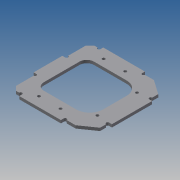
# Autodesk Inventor part: refuerzo interior B
Saved by Autodesk Inventor 2017 (Build 210142000, 142)
## iProperties
Part Number: refuerzo interior B
Material: Genérico
Document SubType Name: Modeling
Designer: Leo
Density: 1 g/cm^3
Appearance: Valor por defecto
Description: Aluminio compuesto routeado CNC
Author: Leo
Autodesk Inventor part; units mm, degrees
ref_plane "YZ Plane" through (0, 0, 0) normal (1, 0, 0) x (0, 1, 0)
ref_plane "XZ Plane" through (0, 0, 0) normal (0, 1, 0) x (-1, 0, 0)
ref_plane "XY Plane" through (0, 0, 0) normal (0, 0, 1) x (1, 0, 0)
sketch "Boceto1" plane through (0, 0, 0) normal (0, 0, 1) x (1, 0, 0)
  line L0 (0, 82.4534) -> (0, -82.4534) construction
  line L1 (-81.8976, 0) -> (81.8976, 0) construction
  line L2 (54.5, 40.5) -> (54.5, 32)
  arc A0 (54.5, 32) -> (54.5, 28) centre (54.5, 30) ccw
  line L3 (54.5, 28) -> (58.5, 28)
  line L4 (58.5, 28) -> (58.5, -28)
  line L5 (58.5, -28) -> (54.5, -28)
  arc A1 (54.5, -28) -> (54.5, -32) centre (54.5, -30) ccw
  line L6 (54.5, -32) -> (54.5, -40.5)
  line L7 (-54.5, 48.5) -> (-54.5, 24)
  arc A2 (-54.5, 20) -> (-54.5, 24) centre (-54.5, 22) ccw
  line L8 (-54.5, 20) -> (-58.5, 20)
  line L9 (-58.5, 20) -> (-58.5, -20)
  line L10 (-58.5, -20) -> (-54.5, -20)
  arc A3 (-54.5, -24) -> (-54.5, -20) centre (-54.5, -22) ccw
  line L11 (-54.5, -24) -> (-54.5, -48.5)
  line L12 (-48.5, 54.5) -> (-44, 54.5)
  line L13 (22, 54.5) -> (34.5, 54.5)
  line L14 (-48.5, -54.5) -> (-44, -54.5)
  line L15 (22, -54.5) -> (34.5, -54.5)
  arc A4 (-44, 54.5) -> (-40, 54.5) centre (-42, 54.5) ccw
  line L16 (-40, 54.5) -> (-40, 58.5)
  line L17 (-40, 58.5) -> (18, 58.5)
  line L18 (18, 58.5) -> (18, 54.5)
  arc A5 (18, 54.5) -> (22, 54.5) centre (20, 54.5) ccw
  arc A6 (-40, -54.5) -> (-44, -54.5) centre (-42, -54.5) ccw
  line L19 (-40, -54.5) -> (-40, -58.5)
  line L20 (-40, -58.5) -> (18, -58.5)
  line L21 (18, -58.5) -> (18, -54.5)
  arc A7 (22, -54.5) -> (18, -54.5) centre (20, -54.5) ccw
  line L22 (-54.5, 48.5) -> (-48.5, 54.5)
  line L23 (54.5, 40.5) -> (34.5, 54.5)
  line L24 (54.5, -40.5) -> (34.5, -54.5)
  line L25 (-48.5, -54.5) -> (-54.5, -48.5)
  line L26 (-39.5, 25) -> (-39.5, -25)
  arc A8 (-39.5, -25) -> (-29.5, -35) centre (-29.5, -25) ccw
  line L27 (-29.5, -35) -> (16.0215, -35)
  arc A9 (16.0215, -35) -> (34.5, -16.5215) centre (16.0215, -16.5215) ccw
  line L28 (34.5, -16.5215) -> (34.5, 16.5215)
  arc A10 (34.5, 16.5215) -> (16.0215, 35) centre (16.0215, 16.5215) ccw
  line L29 (16.0215, 35) -> (-29.5, 35)
  arc A11 (-29.5, 35) -> (-39.5, 25) centre (-29.5, 25) ccw
  circle A12 centre (4, 45) radius 2 projected
  circle A13 centre (-26, 45) radius 2 projected
  line L30 (-37, 36.5) -> (-37, 55.5) construction
  line L31 (15, 55.5) -> (15, 36.5) construction
  circle A14 centre (-26, -45) radius 2 projected
  circle A15 centre (4, -45) radius 2 projected
  line L32 (51.6095, -25) -> (55.9, -25) construction
  circle A16 centre (37.9, 27.5) radius 2 projected
  circle A17 centre (37.9, -27.5) radius 2 projected
  point P0 (0, 0)
  point P1 (0, 0)
  point P2 (54.5, 54.5)
  point P3 (54.5, -54.5)
  point P4 (-54.5, 54.5)
  point P5 (-54.5, -54.5)
  point P6 (54.5, -54.5)
  point P7 (-58.5, 0)
  point P8 (54.5, -54.5)
  point P9 (-39.5, 0)
  point P10 (58.5, 0)
  dimension "d0" = 109
  dimension "d1" = 40
  dimension "d2" = 2
  dimension "d3" = 109
  dimension "d7" = 4
  dimension "d8" = 6
  dimension "d9" = 6
  dimension "d10" = 14
  dimension "d11" = 20
  dimension "d12" = 14
  dimension "d13" = 20
  dimension "d14" = 6
  dimension "d15" = 6
  dimension "d16" = 20
  dimension "d17" = 10
  dimension "d20" = 58
  dimension "d21" = 3
  dimension "d22" = 3
  dimension "d23" = 15
  dimension "d24" = 4
  dimension "d25" = 3
  dimension "d26" = 4
  dimension "d27" = 70
  constraints: 60 end point, 24 point on circle, 23 point on line, 13 tangent, 12 centre point, 12 symmetric about line, 8 perpendicular, 7 equal radius, 6 vertical, 5 horizontal, 5 midpoint, 1 coincident, 1 collinear, 2 other
  measures "d0" distance between parallel lines of L2 L7
  measures "d1" distance of L8.end L9.end
  measures "d2" radius of A2
  measures "d3" distance between parallel lines of L12 L14
  measures "d7" distance between parallel lines of L7 L9
  measures "d8" distance of L7.start point (-54.5, 54.5)
  measures "d9" distance of L12.start point (-54.5, 54.5)
  measures "d10" distance of L2.start point (54.5, 54.5)
  measures "d11" distance of L13.end point (54.5, 54.5)
  measures "d12" distance of L6.end point (54.5, -54.5)
  measures "d13" distance of L15.end point (54.5, -54.5)
  measures "d14" distance of L14.start point (-54.5, -54.5)
  measures "d15" distance of L11.end point (-54.5, -54.5)
  measures "d16" distance between parallel lines of L28 L2
  measures "d17" radius of A11
  measures "d20" distance of L16.end L17.end
  measures "d21" distance between parallel lines of L18 L31
  measures "d22" distance between parallel lines of L16 L30
  measures "d23" distance between parallel lines of L26 L7
  measures "d24" distance between parallel lines of L2 L4
  measures "d25" distance between parallel lines of L5 L32
  measures "d27" distance between parallel lines of L27 L29
extrude "Extrusión1" add sketch "Boceto1" along normal mid plane 4
equation "\"d3\" = d0"
equation "\"d9\" = d8"
equation "\"d12\" = d10"
equation "\"d13\" = d11"
equation "\"d14\" = d8"
equation "\"d15\" = d14"
equation "\"d22\" = d21"
